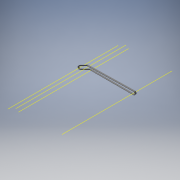
# Autodesk Inventor part: Zahnriemen
Saved by Autodesk Inventor 2019.1 (Build 231200000, 200)
## iProperties
Created: 2018-11-28
Part Number: Zahnriemen
Material: Rubber
Document SubType Name: Modeling
Designer: JochenAlt
Density: 1 g/cm^3
Appearance: Rubber - Black - Version 1.1
CustomPartVersion: 1
Author: JochenAlt
Autodesk Inventor part; units mm, degrees
ref_plane "YZ Plane" through (0, 0, 0) normal (1, 0, 0) x (0, 1, 0)
ref_plane "XZ Plane" through (0, 0, 0) normal (0, 1, 0) x (-1, 0, 0)
ref_plane "XY Plane" through (0, 0, 0) normal (0, 0, 1) x (1, 0, 0)
sketch "Skizzenpfad" plane through (0, 0, 0) normal (0, 0, 1) x (1, 0, 0)
  arc A0 (20.929186, 14.682311) -> (19.564749, 14.341157) centre (21, 11.5) ccw
  arc A1 (143.418533, 9.44913) -> (143.324875, 17.405889) centre (143.413392, 13.428) ccw
  arc A2 (27.997028, 9.299998) -> (26.970103, 9.056529) centre (28, 7) ccw
  arc A3 (-1.794064, 3.551446) -> (1.781665, -3.557682) centre (0, 0) ccw
  line L0 (-1.794064, 3.551446) -> (19.564749, 14.341157)
  line L1 (20.929186, 14.682311) -> (143.324875, 17.405889)
  line L2 (143.418533, 9.44913) -> (27.997028, 9.299998)
  line L3 (26.970103, 9.056529) -> (1.781665, -3.557682)
  constraints: 8 end point, 8 point on circle, 4 centre point
ref_plane "Querschnittsebene" through (19.564749, 14.341157, 0) normal (-0.8925758, -0.4508975, 0) x (0, 0, 1)
ref_plane "Arbeitsebene2" through (21, 11.5, 0) normal (-1, 0, 0) x (0, 0, 1)
ref_plane "Arbeitsebene3" through (143.413392, 13.428, 0) normal (-0.9998999, 0.0141511, 0) x (0, 0, 1)
ref_plane "Arbeitsebene4" through (0, 0, 0) normal (0.9748553, 0.2228388, 0) x (0, 0, 1)
sketch "Querschnitt" plane through (19.564749, 14.341157, 0) normal (-0.8925758, -0.4508975, 0) x (0, 0, 1)
  line L0 (-2, 0.3) -> (2, 0.3)
  line L1 (2, 0.3) -> (2, -0.3)
  line L2 (2, -0.3) -> (-2, -0.3)
  line L3 (-2, -0.3) -> (-2, 0.3)
  line L4 (-2, 0) -> (2, 0) construction
  point P0 (0, 0)
  point P1 (0, 0)
  dimension "d0" = 4
  dimension "d4" = 0.3
  dimension "d5" = 0.3
  constraints: 10 end point, 3 midpoint, 2 parallel, 1 coincident, 1 horizontal, 1 perpendicular, 1 other
  measures "d0" distance between parallel lines of L1 L3
  measures "d4" distance between parallel lines of L2 L4
  measures "d5" distance between parallel lines of L4 L0
sweep "Riemen" add profiles "Querschnitt" path "Skizzenpfad" path curves L3 A3 L0 A0 L1 A1 L2 A2
equation "\"d0\" = da_B"
equation "\"d4\" = da_a"
equation "\"d5\" = da_a2"
equation "\"da_B\" = 4"
equation "\"da_pb\" = 2.5"
equation "\"da_L\" = 317.5"
equation "\"da_a\" = 0.3"
equation "\"da_S\" = 1.5"
equation "\"da_Beta\" = 20deg"
equation "\"da_Ht\" = 0.7"
equation "\"da_H\" = 1.3"
equation "\"da_a2\" = 0.3"
body "Solid1"
